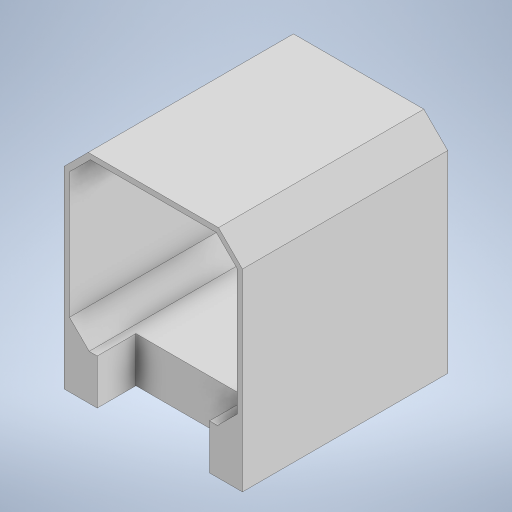
# Autodesk Inventor part: support_moteur_v3
Saved by Autodesk Inventor 2024.2 (Build 282272000, 272)
## iProperties
Created: 2023-12-11
Part Number: support_moteur_v3
Material: Generic
Document SubType Name: Modeling
Designer: adrie
Density: 1 g/cm^3
Appearance: Default
Author: adrie
## iProperties of the stored document support_moteur_v3_Impression 3D.ipt
Created: 2023-12-15
Part Number: support_moteur_v3_Impression 3D
Material: Générique
Document SubType Name: Modeling
Designer: eleves
Density: 1 g/cm^3
Appearance: Par défaut
Author: eleves
Autodesk Inventor part; units mm, degrees
ref_plane "YZ Plane" through (0, 0, 0) normal (1, 0, 0) x (0, 1, 0)
ref_plane "XZ Plane" through (0, 0, 0) normal (0, 1, 0) x (-1, 0, 0)
ref_plane "XY Plane" through (0, 0, 0) normal (0, 0, 1) x (1, 0, 0)
sketch "Sketch1" plane through (0, 0, 0) normal (0, 0, 1) x (1, 0, 0)
  circle A0 centre (-16.8557, -9.8022) radius 17.5002 projected
  circle A1 centre (-1.3556, 5.698) radius 1.5 projected
  circle A2 centre (-32.3556, 5.698) radius 1.5 projected
  circle A3 centre (-1.3556, -25.302) radius 1.5 projected
  circle A4 centre (-32.3556, -25.302) radius 1.5 projected
  line L0 (6.1444, -42.802) -> (-39.8556, -42.802) projected
  line L1 (6.1444, 7.0264) -> (6.1444, -42.802) projected
  line L2 (-39.8556, -42.802) -> (-39.8556, 7.0264) projected
  line L3 (-39.8556, 7.0264) -> (-33.684, 13.198) projected
  line L4 (-33.684, 13.198) -> (-0.0271, 13.198) projected
  line L5 (-0.0271, 13.198) -> (6.1444, 7.0264) projected
  line L6 (-38.5056, 6.4672) -> (-33.1248, 11.848) projected
  line L7 (-0.5863, 11.848) -> (-33.1248, 11.848) projected
  line L8 (-0.5863, 11.848) -> (4.7944, 6.4672) projected
  line L9 (4.7944, 6.4672) -> (4.7944, -26.0712) projected
  line L10 (4.7944, -26.0712) -> (-0.2863, -31.152) projected
  line L11 (-2.3556, -31.152) -> (-31.3556, -31.152) projected
  line L12 (-0.2863, -31.152) -> (-2.3556, -31.152) projected
  line L13 (-38.5056, -26.0712) -> (-33.4248, -31.152) projected
  line L14 (-31.3556, -31.152) -> (-33.4248, -31.152) projected
  line L15 (-38.5056, -26.0712) -> (-38.5056, 6.4672) projected
  point P0 (0, 0)
extrude "Extrusion1" add sketch "Sketch1" along normal blind 5 contours L0 L2 L3 L4 L5 L1 | L6 L7 L8 L9 L10 L12 L11 L14 L13 L15
sketch "Sketch2" plane through (0, 0, 0) normal (0, 0, -1) x (-1, 0, 0)
  line L0 (33.1248, 11.848) -> (0.5863, 11.848) projected
  line L1 (38.5056, 6.4672) -> (33.1248, 11.848) projected
  line L2 (38.5056, -26.0712) -> (38.5056, 6.4672) projected
  line L3 (33.4248, -31.152) -> (38.5056, -26.0712) projected
  line L4 (-6.1444, 7.0264) -> (0.0271, 13.198) projected
  line L5 (-6.1444, -42.802) -> (-6.1444, 7.0264) projected
  line L6 (-4.7944, -26.0712) -> (0.2863, -31.152) projected
  line L7 (-6.1444, 7.0264) -> (0.0271, 13.198) projected
  line L8 (0.0271, 13.198) -> (33.684, 13.198) projected
  line L9 (33.684, 13.198) -> (39.8556, 7.0264) projected
  line L10 (39.8556, 7.0264) -> (39.8556, -42.802) projected
  line L11 (39.8556, -42.802) -> (-6.1444, -42.802) projected
  line L12 (-6.1444, -42.802) -> (-6.1444, 7.0264) projected
  circle A0 centre (16.8557, -9.8022) radius 17.5002 projected
  circle A1 centre (1.3556, 5.698) radius 1.5 projected
  circle A2 centre (32.3556, 5.698) radius 1.5 projected
  circle A3 centre (1.3556, -25.302) radius 1.5 projected
  circle A4 centre (32.3556, -25.302) radius 1.5 projected
  line L13 (0.2863, -31.152) -> (2.3556, -31.152) projected
  line L14 (2.3556, -31.152) -> (31.3556, -31.152) projected
  line L15 (31.3556, -31.152) -> (33.4248, -31.152) projected
  line L16 (33.4248, -31.152) -> (38.5056, -26.0712) projected
  line L17 (0.5863, 11.848) -> (-4.7944, 6.4672) projected
  line L18 (-4.7944, 6.4672) -> (-4.7944, -26.0712) projected
  point P0 (0, 0)
extrude "Extrusion2" add sketch "Sketch2" against normal blind 43 contours L4 L8 L9 L10 L11 L5
sketch "Sketch3" plane through (0, 0, 43) normal (0, 0, 1) x (1, 0, 0)
  line L0 (6.1444, -42.802) -> (6.1444, 7.0264) projected
  line L1 (-2.3556, -42.802) -> (6.1444, -42.802) projected
  line L2 (-2.3556, -42.802) -> (-2.3556, -31.152) projected
  line L3 (4.7944, -26.0712) -> (-0.2863, -31.152) projected
  line L4 (4.7944, 6.4672) -> (4.7944, -26.0712) projected
  line L5 (-39.8556, 7.0264) -> (-39.8556, -42.802) projected
  line L6 (-39.8556, -42.802) -> (6.1444, -42.802) projected
  line L7 (6.1444, -42.802) -> (6.1444, 7.0264) projected
  line L8 (6.1444, 7.0264) -> (-0.0271, 13.198) projected
  line L9 (-0.0271, 13.198) -> (-33.684, 13.198) projected
  line L10 (-33.684, 13.198) -> (-39.8556, 7.0264) projected
  line L11 (-0.2863, -31.152) -> (-33.4248, -31.152) projected
  line L12 (-33.4248, -31.152) -> (-38.5056, -26.0712) projected
  line L13 (-38.5056, -26.0712) -> (-38.5056, 6.4672) projected
  line L14 (-38.5056, 6.4672) -> (-33.1248, 11.848) projected
  line L15 (-33.1248, 11.848) -> (-0.5863, 11.848) projected
  line L16 (-0.5863, 11.848) -> (4.7944, 6.4672) projected
  line L17 (4.7944, 6.4672) -> (4.7944, -26.0712) projected
  line L18 (4.7944, -26.0712) -> (-0.2863, -31.152) projected
  line L19 (-31.3556, -42.802) -> (-31.3556, -31.152) projected
  point P0 (0, 0)
extrude "Extrusion3" add sketch "Sketch3" along normal blind 10 contours L1 L2 L11 L3 L4 L16 L15 L14 L13 L12 L19 L6 L5 L10 L9 L8 L0
sketch "Sketch4" plane through (-39.8556, -42.802, 0) normal (0, -1, 0) x (1, 0, 0)
  line L0 (8.5, 43) -> (37.5, 43) projected
  line L1 (0, 0) -> (46, 0) projected
  line L2 (8.5, 43) -> (8.5, 0) construction
  line L3 (37.5, 43) -> (37.5, 0) construction
  line L4 (8.5, 43) -> (37.5, 0) construction
  line L5 (8.5, 0) -> (37.5, 43) construction
  line L6 (23, 21.5) -> (8.5, 21.5) construction
  line L7 (8.5, 21.5) -> (37.5, 43) construction
  line L8 (8.5, 43) -> (37.5, 21.5) construction
  circle A0 centre (23, 32.25) radius 3.5056
  circle A1 centre (23, 10.75) radius 3.5056
  point P0 (39.8556, 0)
  constraints: 14 end point, 4 midpoint, 2 centre point, 2 perpendicular, 2 point on line, 1 symmetric about line, 1 other
extrude "Extrusion5" cut sketch "Sketch4" against normal blind 9
body "Solid1"
